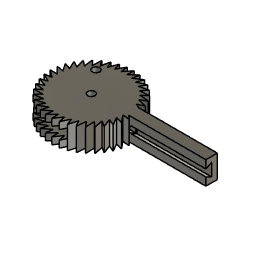
contact (Autodesk Fusion 360 design; units mm, degrees)
Autodesk Fusion 360 part; units mm, degrees
note: some values were not read from the file. Set by a fixed rule: which sketch regions a step uses.
sketch "Esboço1" plane through (0, 0, 0) normal (0, 0, 1) x (1, 0, 0)
  circle A0 centre (0, 0) radius 15
  line L0 (5, 0) -> (30, 0)
  line L1 (30, 0) -> (30, 5)
  line L2 (30, 5) -> (5, 5)
  line L3 (5, 5) -> (5, 0)
  line L4 (-15, 0) -> (-18, 0)
  line L5 (-18, 0) -> (-14.8037, -2.4188)
  dimension "d1" = 30
  dimension "d41" = 3
  constraint coincident A0.centre origin
  constraint horizontal L0
  constraint vertical L1
  constraint horizontal L2
  constraint vertical L3
  constraint coincident A0 L4.start
  constraint horizontal L4
  constraint coincident A0 L5.end
  measures "d1" diameter of A0
  measures "d41" distance of L4.start L4.end
extrude "Extrusão1" add sketch "Esboço1" along normal blind 10 makes body 1
extrude "Extrusão2" add sketch "Esboço1" along normal blind 10 contours A0 L4 L5 bodies 1
pattern_circular "Padrão circular1" count 39 over 360 about axis through (0, 0, 10) along (0, 0, 1) of "Extrusão2"
sketch "Esboço2" plane through (30, 0, 0) normal (1, 0, 0) x (0, 1, 0)
  line L0 (0, 0) -> (5, 0)
  line L1 (5, 0) -> (5, 10)
  line L2 (5, 10) -> (0, 10)
  line L3 (0, 10) -> (0, 0)
  line L4 (0, 6.2) -> (2.0156, 7.2)
  line L5 (2.0156, 7.2) -> (2.0156, 2.8)
  line L6 (2.0156, 2.8) -> (0, 3.8)
  line L7 (0, 6.2) -> (0, 3.8)
  dimension "d8" = 4.4
  dimension "d9" = 2.25
  dimension "d10" = 2.25
  dimension "d11" = 2.4
  dimension "d12" = 3.8
  constraint coincident L3 L4.start
  constraint parallel L3 L5
  constraint coincident L3 L6.end
  measures "d8" distance of L4.end L5.end
  measures "d9" distance of L4.start L4.end
  measures "d10" distance of L5.end L6.end
  measures "d11" distance of L4.start L6.end
  measures "d12" distance of L2.end L4.start
extrude "Extrusão3" cut sketch "Esboço2" against normal blind 19 contours L3 L4 L5 L6 L7 bodies 1
sketch "Esboço3" plane through (0, 0, 10) normal (0, 0, 1) x (-1, 0, 0)
  line L0 (18, 0) -> (14.8178, 2.4081)
  line L1 (15.0122, 0) -> (18, 0)
  line L2 (17.7669, 2.8874) -> (14.2396, 4.7539)
  line L3 (14.8178, 2.4081) -> (17.7669, 2.8874)
  line L4 (17.0737, 5.7) -> (13.2927, 6.9765)
  line L5 (14.2396, 4.7539) -> (17.0737, 5.7)
  line L6 (15.9382, 8.365) -> (12.0014, 9.0185)
  line L7 (13.2927, 6.9765) -> (15.9382, 8.365)
  line L8 (14.39, 10.8134) -> (10.3993, 10.8268)
  line L9 (12.0014, 9.0185) -> (14.39, 10.8134)
  line L10 (12.469, 12.9816) -> (8.5279, 12.3548)
  line L11 (10.3993, 10.8268) -> (12.469, 12.9816)
  line L12 (10.2252, 14.8137) -> (6.4356, 13.5628)
  line L13 (8.5279, 12.3548) -> (10.2252, 14.8137)
  line L14 (7.7165, 16.2621) -> (4.1767, 14.4195)
  line L15 (6.4356, 13.5628) -> (7.7165, 16.2621)
  line L16 (5.0079, 17.2893) -> (1.8095, 14.9028)
  line L17 (4.1767, 14.4195) -> (5.0079, 17.2893)
  line L18 (2.1697, 17.8688) -> (-0.6045, 15)
  line L19 (1.8095, 14.9028) -> (2.1697, 17.8688)
  line L20 (-0.7248, 17.9854) -> (-3.0028, 14.7088)
  line L21 (-0.6045, 15) -> (-0.7248, 17.9854)
  line L22 (-3.6005, 17.6362) -> (-5.3234, 14.0367)
  line L23 (-3.0028, 14.7088) -> (-3.6005, 17.6362)
  line L24 (-5.3234, 14.0367) -> (-6.3829, 16.8303)
  line L25 (-9, 15.5885) -> (-9.4944, 11.6285)
  line L26 (-11.384, 13.9429) -> (-11.2368, 9.9549)
  line L27 (-9.4944, 11.6285) -> (-11.384, 13.9429)
  line L28 (-13.4732, 11.9362) -> (-12.6882, 8.0235)
  line L29 (-11.2368, 9.9549) -> (-13.4732, 11.9362)
  line L30 (-15.2134, 9.6204) -> (-13.8109, 5.8843)
  line L31 (-12.6882, 8.0235) -> (-15.2134, 9.6204)
  line L32 (-16.5596, 7.0554) -> (-14.576, 3.5927)
  line L33 (-13.8109, 5.8843) -> (-16.5596, 7.0554)
  line L34 (-14.576, 3.5927) -> (-17.477, 4.3077)
  line L35 (-15.8671, -5) -> (-13.8109, -5.8843)
  line L36 (-16.5596, -7.0554) -> (-12.6882, -8.0235)
  line L37 (-13.8109, -5.8843) -> (-16.5596, -7.0554)
  line L38 (-15.2134, -9.6204) -> (-11.2368, -9.9549)
  line L39 (-12.6882, -8.0235) -> (-15.2134, -9.6204)
  line L40 (-30, 0) -> (-30, -5)
  line L41 (-30, -5) -> (-15.8671, -5)
  circle A0 centre (0, 0) radius 1.6
  line L42 (-11.2368, -9.9549) -> (-13.4732, -11.9362)
  line L43 (-13.4732, -11.9362) -> (-9.4944, -11.6285)
  line L44 (-9.4944, -11.6285) -> (-11.384, -13.9429)
  line L45 (-11.384, -13.9429) -> (-7.5061, -13.001)
  line L46 (-7.5061, -13.001) -> (-9, -15.5885)
  line L47 (-9, -15.5885) -> (-5.3234, -14.0367)
  line L48 (-5.3234, -14.0367) -> (-6.3829, -16.8303)
  line L49 (-6.3829, -16.8303) -> (-3.0028, -14.7088)
  line L50 (-3.0028, -14.7088) -> (-3.6005, -17.6362)
  line L51 (-3.6005, -17.6362) -> (-0.6045, -15)
  line L52 (-0.6045, -15) -> (-0.7248, -17.9854)
  line L53 (-0.7248, -17.9854) -> (1.8095, -14.9028)
  line L54 (1.8095, -14.9028) -> (2.1697, -17.8688)
  line L55 (2.1697, -17.8688) -> (4.1767, -14.4195)
  line L56 (4.1767, -14.4195) -> (5.0079, -17.2893)
  line L57 (5.0079, -17.2893) -> (6.4356, -13.5628)
  line L58 (6.4356, -13.5628) -> (7.7165, -16.2621)
  line L59 (7.7165, -16.2621) -> (8.5279, -12.3548)
  line L60 (8.5279, -12.3548) -> (10.2252, -14.8137)
  line L61 (10.2252, -14.8137) -> (10.3993, -10.8268)
  line L62 (10.3993, -10.8268) -> (12.469, -12.9816)
  line L63 (12.469, -12.9816) -> (12.0014, -9.0185)
  line L64 (12.0014, -9.0185) -> (14.39, -10.8134)
  line L65 (14.39, -10.8134) -> (13.2927, -6.9765)
  line L66 (-6.3829, 16.8303) -> (-7.5061, 13.001)
  line L67 (-7.5061, 13.001) -> (-9, 15.5885)
  line L68 (-17.477, 4.3077) -> (-14.9635, 1.208)
  line L69 (-14.9635, 1.208) -> (-17.9416, 1.4484)
  line L70 (-17.9416, 1.4484) -> (-16.3178, 0)
  line L71 (-16.3178, 0) -> (-30, 0)
  line L72 (13.2927, -6.9765) -> (15.9382, -8.365)
  line L73 (15.9382, -8.365) -> (14.2396, -4.7539)
  line L74 (14.2396, -4.7539) -> (17.0737, -5.7)
  line L75 (17.0737, -5.7) -> (14.8178, -2.4081)
  line L76 (14.8178, -2.4081) -> (17.7669, -2.8874)
  line L77 (17.7669, -2.8874) -> (15.0122, 0)
  dimension "d15" = 3.2
  constraint coincident A0.centre origin
  measures "d15" diameter of A0
extrude "Extrusão4" cut sketch "Esboço3" against normal blind 10 contours A0 bodies 1
ref_plane "Plano de trabalho1" through (0, 0, 12.125) normal (0, -1, 0) x (0, 0, 1)
ref_plane "Plano de trabalho2" through (0, 25, 12.125) normal (0, -1, 0) x (0, 0, 1)
sketch "Esboço4" plane through (0, 25, 0) normal (0, -1, 0) x (0, 0, 1)
  line L0 (3, -5) -> (7, -5)
  line L1 (7, -5) -> (7, 21.5806)
  line L2 (7, 21.5806) -> (3, 21.5806)
  line L3 (3, 21.5806) -> (3, -5)
  dimension "d20" = 4
  dimension "d21" = 3
  constraint horizontal L0
  constraint vertical L1
  constraint horizontal L2
  constraint vertical L3
  measures "d20" distance of L0.start L0.end
  measures "d21" distance of origin L3
extrude "Extrusão5" cut sketch "Esboço4" along normal blind 45 bodies 1
sketch "Esboço5" plane through (0, 0, 3) normal (0, 0, 1) x (-1, 0, 0)
  line L0 (10.2252, 14.8137) -> (6.4356, 13.5628)
  line L1 (-5, 14.7123) -> (-5, -15.9623)
  circle A0 centre (8, -10) radius 1.6
  line L2 (6.4356, 13.5628) -> (7.7165, 16.2621)
  circle A1 centre (0, 0) radius 1.6
  line L3 (15.0122, 0) -> (18, 0)
  line L4 (18, 0) -> (14.8178, 2.4081)
  line L5 (14.8178, 2.4081) -> (17.7669, 2.8874)
  line L6 (17.7669, 2.8874) -> (14.2396, 4.7539)
  line L7 (14.2396, 4.7539) -> (17.0737, 5.7)
  line L8 (17.0737, 5.7) -> (13.2927, 6.9765)
  line L9 (13.2927, 6.9765) -> (15.9382, 8.365)
  line L10 (15.9382, 8.365) -> (12.0014, 9.0185)
  line L11 (12.0014, 9.0185) -> (14.39, 10.8134)
  line L12 (14.39, 10.8134) -> (10.3993, 10.8268)
  line L13 (10.3993, 10.8268) -> (12.469, 12.9816)
  line L14 (12.469, 12.9816) -> (8.5279, 12.3548)
  line L15 (8.5279, 12.3548) -> (10.2252, 14.8137)
  line L16 (7.7165, 16.2621) -> (4.1767, 14.4195)
  line L17 (-5, -15.9623) -> (-3.0028, -14.7088)
  line L18 (-3.0028, -14.7088) -> (-3.6005, -17.6362)
  line L19 (-3.6005, -17.6362) -> (-0.6045, -15)
  line L20 (-0.6045, -15) -> (-0.7248, -17.9854)
  line L21 (-0.7248, -17.9854) -> (1.8095, -14.9028)
  line L22 (1.8095, -14.9028) -> (2.1697, -17.8688)
  line L23 (2.1697, -17.8688) -> (4.1767, -14.4195)
  line L24 (4.1767, -14.4195) -> (5.0079, -17.2893)
  line L25 (5.0079, -17.2893) -> (6.4356, -13.5628)
  line L26 (6.4356, -13.5628) -> (7.7165, -16.2621)
  line L27 (7.7165, -16.2621) -> (8.5279, -12.3548)
  line L28 (8.5279, -12.3548) -> (10.2252, -14.8137)
  line L29 (10.2252, -14.8137) -> (10.3993, -10.8268)
  line L30 (10.3993, -10.8268) -> (12.469, -12.9816)
  line L31 (12.469, -12.9816) -> (12.0014, -9.0185)
  line L32 (12.0014, -9.0185) -> (14.39, -10.8134)
  line L33 (14.39, -10.8134) -> (13.2927, -6.9765)
  line L34 (4.1767, 14.4195) -> (5.0079, 17.2893)
  line L35 (5.0079, 17.2893) -> (1.8095, 14.9028)
  line L36 (1.8095, 14.9028) -> (2.1697, 17.8688)
  line L37 (2.1697, 17.8688) -> (-0.6045, 15)
  line L38 (-0.6045, 15) -> (-0.7248, 17.9854)
  line L39 (-0.7248, 17.9854) -> (-3.0028, 14.7088)
  line L40 (13.2927, -6.9765) -> (15.9382, -8.365)
  line L41 (15.9382, -8.365) -> (14.2396, -4.7539)
  line L42 (14.2396, -4.7539) -> (17.0737, -5.7)
  line L43 (17.0737, -5.7) -> (14.8178, -2.4081)
  line L44 (14.8178, -2.4081) -> (17.7669, -2.8874)
  line L45 (17.7669, -2.8874) -> (15.0122, 0)
  line L46 (-3.0028, 14.7088) -> (-3.6005, 17.6362)
  line L47 (-3.6005, 17.6362) -> (-5, 14.7123)
  point P0 (0, 0)
  point P1 (0, 0)
  point P2 (0, 0)
  point P3 (0, 0)
  point P4 (0, 0)
  point P5 (0, 0)
  point P6 (0, 0)
  point P7 (0, 0)
  point P8 (0, 0)
  point P9 (0, 0)
  point P10 (0, 0)
  point P11 (0, 0)
  point P12 (0, 0)
  point P13 (0, 0)
  point P14 (0, 0)
  point P15 (0, 0)
  point P16 (0, 0)
  point P17 (0, 0)
  point P18 (0, 0)
  point P19 (0, 0)
  point P20 (0, 0)
  point P21 (0, 0)
  point P22 (0, 0)
  point P23 (0, 0)
  point P24 (0, 0)
  point P25 (0, 0)
  point P26 (0, 0)
  point P27 (0, 0)
  point P28 (0, 0)
  point P29 (0, 0)
  point P30 (0, 0)
  point P31 (0, 0)
  point P32 (0, 0)
  point P33 (0, 0)
  point P34 (0, 0)
  point P35 (0, 0)
  point P36 (0, 0)
  point P37 (0, 0)
  point P38 (0, 0)
  point P39 (0, 0)
  point P40 (0, 0)
  point P41 (0, 0)
  point P42 (0, 0)
  point P43 (0, 0)
  point P44 (0, 0)
  point P45 (0, 0)
  point P46 (0, 0)
  point P47 (0, 0)
  point P48 (0, 0)
  point P49 (0, 0)
  point P50 (0, 0)
  point P51 (0, 0)
  point P52 (0, 0)
  point P53 (0, 0)
  point P54 (0, 0)
  point P55 (0, 0)
  point P56 (0, 0)
  point P57 (0, 0)
  point P58 (0, 0)
  point P59 (0, 0)
  point P60 (0, 0)
  point P61 (0, 0)
  dimension "d24" = 3.2
  measures "d24" diameter of A0
extrude "Extrusão6" cut sketch "Esboço5" against normal blind 6 contours A0 bodies 1
extrude "Extrusão7" cut sketch "Esboço5" along normal blind 7 contours A0 bodies 1
copy_body "Corpo -> Componente1" bodies 1 removing the originals makes body 2 in component "Component"
sketch "Esboço6" plane through (30, 0, 0) normal (1, 0, 0) x (0, 1, 0)
  line L0 (0, 6.2) -> (2.0156, 7.2)
  line L1 (2.0156, 7.2) -> (2.0156, 2.8)
  line L2 (2.0156, 2.8) -> (0, 3.8)
  line L3 (0, 3.8) -> (0, 0)
  line L4 (0, 0) -> (5, 0)
  line L5 (5, 0) -> (5, 10)
  line L6 (5, 10) -> (0, 10)
  line L7 (0.2342, 6.2703) -> (2.2498, 7.2703)
  line L8 (2.2498, 7.2703) -> (2.2498, 2.8703)
  line L9 (2.2498, 2.8703) -> (0, 2.8407)
  line L10 (0.2342, 6.2703) -> (0, 2.8407)
  line L11 (0, 10) -> (0, 6.2)
  dimension "d31" = 2.25
  dimension "d32" = 4.4
  dimension "d33" = 2.25
  dimension "d34" = 0.2445
  constraint parallel L0 L7
  constraint coincident L3 L9.end
  measures "d31" distance of L7.start L7.end
  measures "d32" distance of L7.end L8.end
  measures "d33" distance of L8.end L9.end
  measures "d34" distance of L0.start L7.start
extrude "Extrusão2'" add 1 faces at (11, 1.3437, 5.4) along direction (1, 0, 0) blind 3.66 on bodies 2 bodies 2 in component "Component"
extrude "Extrusão3'" add 1 faces at (30, 4.0052, 4.2667) along direction (1, 0, 0) blind 20 on bodies 2 bodies 2 in component "Component"
scale "Escala3" factor 0.7 about (16.3178, 0, 6.2) bodies 2 in component "Component"
scale "Escala4" factor 1.14 about (16.3178, 0, 6.2) bodies 2 in component "Component"
sketch "Esboço7" plane through (43.1962, 0, 0) normal (1, 0, 0) x (0, 1, 0)
  line L0 (0, 6.2) -> (1.6084, 6.998)
  line L1 (1.6084, 6.998) -> (1.6084, 3.4868)
  line L2 (1.6084, 3.4868) -> (0, 4.2848)
  line L3 (0, 4.2848) -> (0, 1.2524)
  line L4 (0, 1.2524) -> (3.99, 1.2524)
  line L5 (3.99, 1.2524) -> (3.99, 9.2324)
  line L6 (3.99, 9.2324) -> (0, 9.2324)
  line L7 (0, 9.2324) -> (0, 6.2)
  line L8 (0, 6.4424) -> (2.0156, 7.4424)
  line L9 (2.0156, 7.4424) -> (2.0156, 3.0424)
  line L10 (2.0156, 3.0424) -> (0, 4.0424)
  line L11 (0, 6.4424) -> (0, 4.0424)
  dimension "d44" = 2.25
  dimension "d45" = 4.4
  dimension "d46" = 2.25
  dimension "d47" = 2.79
  constraint parallel L0 L8
  constraint vertical L9
  constraint coincident L3 L10.end
  constraint parallel L3 L11
  measures "d44" distance of L8.start L8.end
  measures "d45" distance of L8.end L9.end
  measures "d46" distance of L9.end L10.end
  measures "d47" distance of L6.end L8.start
extrude "Extrusão4'" cut sketch "Esboço7" against normal blind 26 contours L0 L1 L2 L3 L7 L8 L9 L10 L11 bodies 2 in component "Component"
component "Component" placed x (1, 0, 0) y (0, 1, 0) z (0, 0, 1) at (0, 0, 0)
